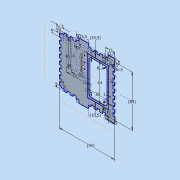
# Autodesk Inventor part: Top_plate
Saved by Autodesk Inventor 2015 (Build 190159000, 159)
## iProperties
Created: 2015-01-31
Part Number: Top_plate
Material: Wood (Birch)
Document SubType Name: Modeling
Designer: Openlab
Density: 0.55 g/cm^3
Appearance: Polycarbonate - Clear
Author: Openlab
Autodesk Inventor part; units mm, degrees
ref_plane "YZ Plane" through (0, 0, 0) normal (1, 0, 0) x (0, 1, 0)
ref_plane "XZ Plane" through (0, 0, 0) normal (0, 1, 0) x (-1, 0, 0)
ref_plane "XY Plane" through (0, 0, 0) normal (0, 0, 1) x (1, 0, 0)
sketch "Sketch1" plane through (0, 0, 0) normal (0, 1, 0) x (-1, 0, 0)
  line L0 (46, -10.5) -> (10, -10.5)
  line L1 (10, -10.5) -> (10, -74.5)
  line L2 (10, -74.5) -> (46, -74.5)
  line L3 (46, -74.5) -> (46, -10.5)
  line L4 (39, -13.5) -> (17, -13.5)
  line L5 (13, -17.5) -> (13, -67.5)
  line L6 (17, -71.5) -> (39, -71.5)
  line L7 (43, -67.5) -> (43, -17.5)
  line L8 (-0.7624, -103.1576) -> (89.2376, -103.1576) construction
  line L9 (117.4263, -3.5737) -> (117.4263, -83.5737) construction
  line L10 (0, 0) -> (0, -5)
  line L11 (0, -5) -> (3, -5)
  line L12 (3, -5) -> (3, -10)
  line L13 (3, -10) -> (0, -10)
  line L14 (0, -10) -> (0, -15)
  line L15 (0, -15) -> (3, -15)
  line L16 (3, -15) -> (3, -20)
  line L17 (3, -20) -> (0, -20)
  line L18 (0, -20) -> (0, -25)
  line L19 (0, -25) -> (3, -25)
  line L20 (3, -25) -> (3, -30)
  line L21 (3, -30) -> (0, -30)
  line L22 (0, -30) -> (0, -35)
  line L23 (0, -35) -> (3, -35)
  line L24 (3, -35) -> (3, -40)
  line L25 (3, -40) -> (0, -40)
  line L26 (0, -40) -> (0, -45)
  line L27 (0, -45) -> (3, -45)
  line L28 (3, -45) -> (3, -50)
  line L29 (3, -50) -> (0, -50)
  line L30 (0, -50) -> (0, -55)
  line L31 (0, -55) -> (3, -55)
  line L32 (3, -55) -> (3, -60)
  line L33 (3, -60) -> (0, -60)
  line L34 (0, -60) -> (0, -65)
  line L35 (0, -65) -> (3, -65)
  line L36 (3, -65) -> (3, -70)
  line L37 (3, -70) -> (0, -70)
  line L38 (0, -70) -> (0, -75)
  line L39 (0, -75) -> (3, -75)
  line L40 (3, -75) -> (3, -80)
  line L41 (11.5, 0) -> (15, 0)
  line L42 (15, 0) -> (15, -3)
  line L43 (15, -3) -> (20, -3)
  line L44 (20, -3) -> (20, 0)
  line L45 (20, 0) -> (25, 0)
  line L46 (25, -3) -> (30, -3)
  line L47 (30, 0) -> (35, 0)
  line L48 (30, -3) -> (30, 0)
  line L49 (25, 0) -> (25, -3)
  line L50 (35, -3) -> (40, -3)
  line L51 (40, 0) -> (44.5, 0)
  line L52 (40, -3) -> (40, 0)
  line L53 (35, 0) -> (35, -3)
  line L54 (60, 0) -> (65, 0)
  line L55 (65, -3) -> (70, -3)
  line L56 (70, 0) -> (75, 0)
  line L57 (70, -3) -> (70, 0)
  line L58 (65, 0) -> (65, -3)
  line L59 (75, -3) -> (80, -3)
  line L60 (80, 0) -> (85, 0)
  line L61 (80, -3) -> (80, 0)
  line L62 (75, 0) -> (75, -3)
  line L63 (90, -3) -> (90, -5)
  line L64 (90, -5) -> (93, -5)
  line L65 (90, -15) -> (93, -15)
  line L66 (93, -5) -> (93, -10)
  line L67 (93, -10) -> (90, -10)
  line L68 (90, -10) -> (90, -15)
  line L69 (90, -25) -> (93, -25)
  line L70 (93, -15) -> (93, -20)
  line L71 (93, -20) -> (90, -20)
  line L72 (90, -20) -> (90, -25)
  line L73 (90, -35) -> (93, -35)
  line L74 (93, -25) -> (93, -30)
  line L75 (93, -30) -> (90, -30)
  line L76 (90, -30) -> (90, -35)
  line L77 (90, -45) -> (93, -45)
  line L78 (93, -35) -> (93, -40)
  line L79 (93, -40) -> (90, -40)
  line L80 (90, -40) -> (90, -45)
  line L81 (90, -55) -> (93, -55)
  line L82 (93, -45) -> (93, -50)
  line L83 (93, -50) -> (90, -50)
  line L84 (90, -50) -> (90, -55)
  line L85 (93, -55) -> (93, -60)
  line L86 (93, -60) -> (90, -60)
  line L87 (90, -60) -> (90, -65)
  line L88 (3, -80) -> (0, -80)
  line L89 (0, -80) -> (0, -85)
  line L90 (11.5, -85) -> (15, -85)
  line L91 (15, -85) -> (15, -82)
  line L92 (15, -82) -> (20, -82)
  line L93 (20, -82) -> (20, -85)
  line L94 (20, -85) -> (25, -85)
  line L95 (25, -82) -> (30, -82)
  line L96 (30, -85) -> (35, -85)
  line L97 (30, -82) -> (30, -85)
  line L98 (25, -85) -> (25, -82)
  line L99 (35, -82) -> (40, -82)
  line L100 (40, -85) -> (44.5, -85)
  line L101 (40, -82) -> (40, -85)
  line L102 (35, -85) -> (35, -82)
  line L103 (60, -85) -> (65, -85)
  line L104 (65, -82) -> (70, -82)
  line L105 (70, -85) -> (75, -85)
  line L106 (70, -82) -> (70, -85)
  line L107 (65, -85) -> (65, -82)
  line L108 (75, -82) -> (80, -82)
  line L109 (80, -85) -> (85, -85)
  line L110 (80, -82) -> (80, -85)
  line L111 (75, -85) -> (75, -82)
  line L112 (90, -65) -> (93, -65)
  line L113 (93, -65) -> (93, -70)
  line L114 (93, -70) -> (90, -70)
  line L115 (90, -70) -> (90, -75)
  line L116 (90, -75) -> (93, -75)
  line L117 (93, -75) -> (93, -80)
  line L118 (93, -80) -> (90, -80)
  line L119 (-8, -42.5) -> (-32, -42.5) construction
  line L120 (85, -85) -> (85, -82)
  line L121 (85, -82) -> (90, -82)
  line L122 (85, 0) -> (85, -3)
  line L123 (85, -3) -> (90, -3)
  line L124 (90, -82) -> (90, -80)
  line L125 (50, -42.5) -> (84, -42.5) construction
  circle A0 centre (50, -36) radius 3 construction
  line L126 (81, -48) -> (46, -48) construction
  line L127 (72.771, -46.18) -> (54.229, -46.18) construction
  circle A1 centre (50, -36) radius 2.5 construction
  line L128 (67.5, -8) -> (59.5, -8) construction
  line L129 (67.5, -3) -> (67.5, -8) construction
  line L130 (59.5, -8) -> (59.5, -3) construction
  circle A2 centre (50, -26) radius 2.5 construction
  circle A3 centre (50, -26) radius 3 construction
  line L131 (63.5, 13.6319) -> (63.5, -36.0508) construction
  line L132 (46, -48) -> (46, -3) construction
  line L133 (81, -3) -> (81, -48) construction
  line L134 (54.229, -46.18) -> (54.229, -3) construction
  line L135 (72.771, -3) -> (72.771, -46.18) construction
  circle A4 centre (50, -16) radius 2.5 construction
  circle A5 centre (50, -16) radius 3 construction
  line L136 (46, -3) -> (81, -3) construction
  line L137 (54.229, -3) -> (72.771, -3) construction
  line L138 (59.5, -3) -> (67.5, -3) construction
  arc A6 (17, -13.5) -> (13, -17.5) centre (17, -17.5) ccw
  arc A7 (13, -67.5) -> (17, -71.5) centre (17, -67.5) ccw
  arc A8 (43, -17.5) -> (39, -13.5) centre (39, -17.5) ccw
  arc A9 (39, -71.5) -> (43, -67.5) centre (39, -67.5) ccw
  line L139 (44.5, 6) -> (44.5, -102) construction
  line L140 (44.5, -85) -> (44.5, -90) construction
  line L141 (44.5, -85) -> (44.5, -90)
  line L142 (44.5, -90) -> (60, -90)
  line L143 (60, -90) -> (60, -85)
  line L144 (44.5, 0) -> (44.5, 5)
  line L145 (60, 5) -> (60, 0)
  line L146 (44.5, 5) -> (60, 5)
  line L147 (11.5, -6) -> (11.5, -76.5659) construction
  line L148 (11.5, -85) -> (11.5, -90)
  line L149 (11.5, -90) -> (0, -90)
  line L150 (0, -90) -> (0, -85)
  line L151 (11.5, 0) -> (11.5, 5)
  line L152 (11.5, 5) -> (0, 5)
  line L153 (0, 5) -> (0, 0)
  point P0 (85, -77)
  point P1 (85, -8)
  point P2 (8, -8)
  point P3 (8, -77)
  dimension "d0" = 36
  dimension "d1" = 64
  dimension "d15" = 3
  dimension "d17" = 3
  dimension "d18" = 3
  dimension "d19" = 15
  dimension "d20" = 5
  dimension "d21" = 3
  dimension "d22" = 5
  dimension "d23" = 3
  dimension "d24" = 3
  dimension "d25" = 5
  dimension "d26" = 15
  dimension "d27" = 7
  dimension "d28" = 5
  dimension "d35" = 3
  dimension "d36" = 3
  dimension "d37" = 5
  dimension "d38" = 5
  dimension "d39" = 85
  dimension "d40" = 5
  dimension "d41" = 5
  dimension "d42" = 5
  dimension "d43" = 5
  dimension "d101" = 10
  dimension "d102" = 10
  dimension "d103" = 4
  dimension "d104" = 12
  dimension "d105" = 18.542
  dimension "d106" = 35
  dimension "d107" = 45
  dimension "d108" = 8
  dimension "d109" = 5
  dimension "d110" = 43.18
  dimension "d118" = 8
  dimension "d120" = 5
  dimension "d121" = 5
  dimension "d122" = 15.5
  dimension "d124" = 1.5
  dimension "d125" = 1.5
  dimension "d126" = 5
  dimension "d127" = 11.5
  dimension "d128" = 5
  dimension "d129" = 3.5
  dimension "d130" = 3.5
  dimension "d131" = 5
  dimension "d132" = 10.5
  dimension "d133" = 10.5
  dimension "d134" = 93
  constraints: 308 end point, 104 perpendicular, 54 equal length, 42 collinear, 22 point on line, 11 coincident, 10 centre point, 9 vertical, 8 horizontal, 8 point on circle, 8 tangent, 6 vertical alignment, 4 horizontal alignment, 6 other
  measures "d0" distance of L2.end L1.end
  measures "d1" distance of L1.end L0.end
  measures "d15" distance between parallel lines of L0 L4
  measures "d17" distance between parallel lines of L1 L5
  measures "d18" distance between parallel lines of L2 L6
  measures "d19" distance of L10.start L41.end
  measures "d20" distance of L42.end L43.end
  measures "d21" distance of L41.end L42.end
  measures "d22" distance of L10.start L10.end
  measures "d23" distance of L10.end L11.end
  measures "d24" distance of L90.end L91.end
  measures "d25" distance of L91.end L92.end
  measures "d26" distance of L89.end L90.end
  measures "d27" distance between parallel lines of L24 L1
  measures "d28" distance of L64.end L66.end
  measures "d35" distance between parallel lines of L7 L3
  measures "d36" distance of L63.end L64.end
  measures "d37" distance between parallel lines of L60 L64
  measures "d38" distance between parallel lines of L109 L118
  measures "d39" distance between parallel lines of L41 L90
  measures "d40" distance from line of L121 point (85, -77)
  measures "d41" distance from line of L115 point (85, -77)
  measures "d42" distance from line of L43 point (8, -8)
  measures "d43" distance from line of L12 point (8, -8)
  measures "d101" distance of A3.centre A1.centre
  measures "d102" distance of A4.centre A3.centre
  measures "d103" distance from line of L132 A4.centre
  measures "d104" distance from line of L126 A1.centre
  measures "d105" distance of L127.start L134.start
  measures "d106" distance of L126.start L132.start
  measures "d107" distance of L136.end L126.start
  measures "d108" distance of L128.start L128.end
  measures "d109" distance of L128.end L138.start
  measures "d110" distance of L137.end L127.start
  measures "d118" diameter of A6
  measures "d120" distance of L142.end L103.start
  measures "d121" distance of L145.start L54.start
  measures "d122" distance of L144.end L145.start
  measures "d124" distance between parallel lines of L7 L139
  measures "d125" distance between parallel lines of L5 L147
  measures "d126" distance of L152.end L10.start
  measures "d127" distance of L151.end L152.end
  measures "d128" distance of L149.end L89.end
  measures "d129" distance of L41.start L41.end
  measures "d130" distance of L90.start L90.end
  measures "d131" distance of L54.start L54.end
  measures "d132" distance between parallel lines of L47 L0
  measures "d133" distance between parallel lines of L96 L2
  measures "d134" distance between parallel lines of L113 L38
extrude "Extrusion1" add sketch "Sketch1" along normal blind 3 contours L3 L2 L1 L0 | L153 L152 L151 L41 L42 L43 L44 L45 L49 L46 L48 L47 L53 L50 L52 L51 L144 L146 L145 L54 L58 L55 L57 L56 L62 L59 L61 L60 L122 L123 L63 L64 L66 L67 L68 L65 L70 L71 L72 L69 L74 L75 L76 L73 L78 L79 L80 L77 L82 L83 L84 L81 L85 L86 L87 L112 L113 L114 L115 L116 L117 L118 L124 L121 L120 L109 L110 L108 L111 L105 L106 L104 L107 L103 L143 L142 L141 L100 L101 L99 L102 L96 L97 L95 L98 L94 L93 L92 L91 L90 L148 L149 L150 L89 L88 L40 L39 L38 L37 L36 L35 L34 L33 L32 L31 L30 L29 L28 L27 L26 L25 L24 L23 L22 L21 L20 L19 L18 L17 L16 L15 L14 L13 L12 L11 L10
hole "Hole1" at (-85, 0, -77) at (-85, 0, -8) at (-8, 0, -8) at (-8, 0, -77) direction (0, 1, 0) diameter 3 end through all
hole "Hole2" at (-50, 0, -36) at (-50, 0, -26) at (-50, 0, -16) direction (0, 1, 0) diameter 5 end through all
equation "\"d21\" = x"
equation "\"d23\" = x"
equation "\"d24\" = x"
equation "\"d36\" = x"
equation "\"x\" = 3"
body "Solid1"
